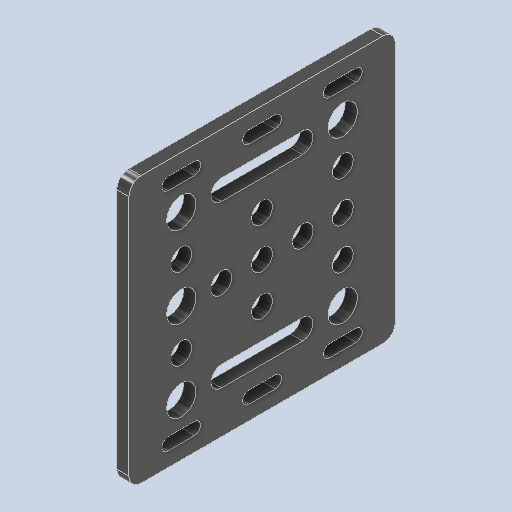
# Autodesk Inventor part: HCMUTE-CDT23-OP_BASE-PLATE
Saved by Autodesk Inventor 2023 (Build 270158000, 158)
## iProperties
Created: 2023-11-14
Part Number: HCMUTE-CDT23-OP_BASE-PLATE
Material: Aluminum 6061
Document SubType Name: Sheet Metal
Designer: havie
Density: 2.7 g/cm^3
Sheet Metal Rule: Default_mm
Appearance: Dark Gray
Author: havie
Autodesk Inventor part; units mm, degrees
ref_plane "YZ Plane" through (0, 0, 0) normal (1, 0, 0) x (0, 1, 0)
ref_plane "XZ Plane" through (0, 0, 0) normal (0, 1, 0) x (-1, 0, 0)
ref_plane "XY Plane" through (0, 0, 0) normal (0, 0, 1) x (1, 0, 0)
sketch "Sketch1" plane through (0, 0, 0) normal (1, 0, 0) x (0, 1, 0)
  line L0 (32.75, 32.75) -> (-32.75, 32.75)
  line L1 (-32.75, 32.75) -> (-32.75, -32.75)
  line L2 (-32.75, -32.75) -> (32.75, -32.75)
  line L3 (32.75, -32.75) -> (32.75, 32.75)
  line L4 (32.75, 32.75) -> (-32.75, -32.75) construction
  line L5 (-32.75, 32.75) -> (32.75, -32.75) construction
  circle A0 centre (0, 0) radius 2.55
  circle A1 centre (0, 10) radius 2.55
  circle A2 centre (0, -10) radius 2.55
  circle A3 centre (0, -19.85) radius 2.55
  circle A4 centre (0, 19.85) radius 3.6
  circle A5 centre (10, 0) radius 2.55
  circle A6 centre (-10, 0) radius 2.55
  circle A7 centre (-10, -19.85) radius 2.55
  circle A8 centre (10, -19.85) radius 2.55
  circle A9 centre (-10, 19.85) radius 2.55
  circle A10 centre (10, 19.85) radius 2.55
  circle A11 centre (20, 19.85) radius 3.6
  circle A12 centre (-20, 19.85) radius 3.6
  circle A13 centre (19.85, -19.85) radius 3.6
  circle A14 centre (-19.85, -19.85) radius 3.6
  line L6 (27.7, 16.6) -> (27.7, 23.1) construction
  line L7 (26.2, 16.6) -> (26.2, 23.1)
  line L8 (29.2, 23.1) -> (29.2, 16.6)
  arc A15 (26.2, 16.6) -> (29.2, 16.6) centre (27.7, 16.6) ccw
  arc A16 (29.2, 23.1) -> (26.2, 23.1) centre (27.7, 23.1) ccw
  line L9 (27.7, 3.25) -> (27.7, -3.25) construction
  line L10 (26.2, 3.25) -> (26.2, -3.25)
  line L11 (29.2, -3.25) -> (29.2, 3.25)
  arc A17 (29.2, 3.25) -> (26.2, 3.25) centre (27.7, 3.25) ccw
  arc A18 (26.2, -3.25) -> (29.2, -3.25) centre (27.7, -3.25) ccw
  line L12 (27.7, -16.6) -> (27.7, -23.1) construction
  line L13 (26.2, -16.6) -> (26.2, -23.1)
  line L14 (29.2, -23.1) -> (29.2, -16.6)
  arc A19 (29.2, -16.6) -> (26.2, -16.6) centre (27.7, -16.6) ccw
  arc A20 (26.2, -23.1) -> (29.2, -23.1) centre (27.7, -23.1) ccw
  line L15 (-27.7, 16.6) -> (-27.7, 23.1) construction
  line L16 (-26.2, 16.6) -> (-26.2, 23.1)
  line L17 (-29.2, 23.1) -> (-29.2, 16.6)
  arc A21 (-29.2, 16.6) -> (-26.2, 16.6) centre (-27.7, 16.6) ccw
  arc A22 (-26.2, 23.1) -> (-29.2, 23.1) centre (-27.7, 23.1) ccw
  line L18 (-27.7, 3.25) -> (-27.7, -3.25) construction
  line L19 (-29.2, 3.25) -> (-29.2, -3.25)
  line L20 (-26.2, -3.25) -> (-26.2, 3.25)
  arc A23 (-26.2, 3.25) -> (-29.2, 3.25) centre (-27.7, 3.25) ccw
  arc A24 (-29.2, -3.25) -> (-26.2, -3.25) centre (-27.7, -3.25) ccw
  line L21 (-27.7, -16.6) -> (-27.7, -23.1) construction
  line L22 (-26.2, -16.6) -> (-26.2, -23.1)
  line L23 (-29.2, -23.1) -> (-29.2, -16.6)
  arc A25 (-26.2, -16.6) -> (-29.2, -16.6) centre (-27.7, -16.6) ccw
  arc A26 (-29.2, -23.1) -> (-26.2, -23.1) centre (-27.7, -23.1) ccw
  line L24 (-19.85, 10) -> (-19.85, -10) construction
  line L25 (-17.35, 10) -> (-17.35, -10)
  line L26 (-22.35, -10) -> (-22.35, 10)
  arc A27 (-17.35, 10) -> (-22.35, 10) centre (-19.85, 10) ccw
  arc A28 (-22.35, -10) -> (-17.35, -10) centre (-19.85, -10) ccw
  line L27 (19.85, 10) -> (19.85, -10) construction
  line L28 (17.35, 10) -> (17.35, -10)
  line L29 (22.35, -10) -> (22.35, 10)
  arc A29 (22.35, 10) -> (17.35, 10) centre (19.85, 10) ccw
  arc A30 (17.35, -10) -> (22.35, -10) centre (19.85, -10) ccw
  point P0 (27.7, 19.85)
  point P1 (27.7, 0)
  point P2 (27.7, -19.85)
  point P3 (-27.7, 19.85)
  point P4 (-27.7, 0)
  point P5 (-27.7, -19.85)
  point P6 (-19.85, 0)
  point P7 (19.85, 0)
  dimension "d4" = 65.5
  dimension "d5" = 65.5
  dimension "d6" = 5.1
  dimension "d7" = 5.1
  dimension "d8" = 5.1
  dimension "d9" = 5.1
  dimension "d10" = 22.75
  dimension "d11" = 42.75
  dimension "d12" = 52.6
  dimension "d13" = 7.2
  dimension "d14" = 12.9
  dimension "d15" = 5.1
  dimension "d16" = 5.1
  dimension "d17" = 22.75
  dimension "d18" = 42.75
  dimension "d19" = 5.1
  dimension "d20" = 5.1
  dimension "d21" = 5.1
  dimension "d22" = 5.1
  dimension "d23" = 7.2
  dimension "d24" = 7.2
  dimension "d25" = 12.75
  dimension "d26" = 52.75
  dimension "d27" = 7.2
  dimension "d28" = 7.2
  dimension "d30" = 5.05
  dimension "d31" = 5.05
  dimension "d33" = 6.5
  dimension "d34" = 3
  dimension "d35" = 6.5
  dimension "d36" = 6.5
  dimension "d37" = 3
  dimension "d38" = 3
  dimension "d39" = 3
  dimension "d40" = 3
  dimension "d41" = 20
  dimension "d42" = 5
  dimension "d43" = 20
  dimension "d44" = 5
  measures "d4" distance of L0.end L1.end
  measures "d5" distance of L1.end L2.end
  measures "d6" diameter of A0
  measures "d7" diameter of A1
  measures "d8" diameter of A2
  measures "d9" diameter of A3
  measures "d10" distance from line of L0 A1.centre
  measures "d11" distance from line of L0 A2.centre
  measures "d12" distance from line of L0 A3.centre
  measures "d13" diameter of A4
  measures "d14" distance from line of L0 A4.centre
  measures "d15" diameter of A6
  measures "d16" diameter of A5
  measures "d17" distance from line of L3 A5.centre
  measures "d18" distance from line of A6.centre L3
  measures "d19" diameter of A8
  measures "d20" diameter of A7
  measures "d21" diameter of A9
  measures "d22" diameter of A10
  measures "d23" diameter of A12
  measures "d24" diameter of A11
  measures "d25" distance from line of L3 A11.centre
  measures "d26" distance from line of L3 A12.centre
  measures "d27" diameter of A13
  measures "d28" diameter of A14
  measures "d30" distance from line of point (27.7, 19.85) L3
  measures "d31" distance between parallel lines of L15 L1
  measures "d33" distance of L8.start L8.end
  measures "d34" distance between parallel lines of L7 L8
  measures "d35" distance of L11.start L11.end
  measures "d36" distance of L14.start L14.end
  measures "d37" distance between parallel lines of L13 L14
  measures "d38" distance between parallel lines of L17 L16
  measures "d39" distance between parallel lines of L19 L20
  measures "d40" distance between parallel lines of L23 L22
  measures "d41" distance of L26.start L26.end
  measures "d42" distance between parallel lines of L26 L25
  measures "d43" distance of L28.start L28.end
  measures "d44" distance between parallel lines of L28 L29
extrude "Plate1" add sketch "Sketch1" along normal mid plane 3
fillet "Corner Round1" radius 3 4 edges at (0, 32.75, 32.75) (0, 32.75, -32.75) (0, -32.75, -32.75) (0, -32.75, 32.75)
equation "\"d5\" = d4"
equation "\"d7\" = d6"
equation "\"d8\" = d6"
equation "\"d9\" = d8"
equation "\"d15\" = d6"
equation "\"d16\" = d6"
equation "\"d19\" = d9"
equation "\"d20\" = d9"
equation "\"d21\" = d7"
equation "\"d22\" = d21"
equation "\"d23\" = d13"
equation "\"d24\" = d23"
equation "\"d27\" = d23"
equation "\"d28\" = d23"
equation "\"d45\" = Thickness"
equation "\"BendRadius\" = Thickness"
equation "\"BendReliefWidth\" = Thickness"
equation "\"BendReliefDepth\" = 0.5 * Thickness"
equation "\"CornerReliefSize\" = 4 * Thickness"
equation "\"MinimumRemnant\" = 2 * Thickness"
equation "\"TransitionRadius\" = BendRadius"
equation "\"JacobiRadiusSize\" = BendRadius"
equation "\"GapSize\" = Thickness"
equation "\"Thickness\" = 3"
body "Solid1"
